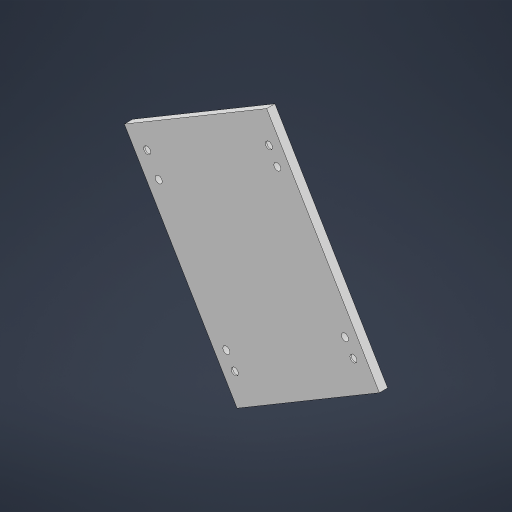
# Autodesk Inventor part: ThirdPlate
Saved by Autodesk Inventor 2024.2 (Build 282272000, 272)
## iProperties
Created: 2023-12-27
Part Number: ThirdPlate
Material: 一般
Document SubType Name: Modeling
Designer: Hanaoka
Density: 1 g/cm^3
Appearance: 既定
Author: Hanaoka
Autodesk Inventor part; units mm, degrees
ref_plane "YZ Plane" through (0, 0, 0) normal (1, 0, 0) x (0, 1, 0)
ref_plane "XZ Plane" through (0, 0, 0) normal (0, 1, 0) x (-1, 0, 0)
ref_plane "XY Plane" through (0, 0, 0) normal (0, 0, 1) x (1, 0, 0)
sketch "スケッチ1" plane through (0, 0, 0) normal (0, 0, 1) x (1, 0, 0)
  line L0 (9.406, -6.0438) -> (-42.1785, -36.6875)
  line L1 (-42.1785, -36.6875) -> (-83.0369, 32.0918)
  line L2 (-83.0369, 32.0918) -> (-31.4524, 62.7355)
  line L3 (-31.4524, 62.7355) -> (9.406, -6.0438)
  circle A0 centre (-42.9871, -25.5365) radius 1.3 projected
  circle A1 centre (-74.7819, 27.9857) radius 1.3 projected
  circle A2 centre (-30.6438, 51.5845) radius 1.3 projected
  circle A3 centre (0, 0) radius 1.3 projected
  line L4 (-30.6438, 51.5845) -> (-26.3451, 54.1381) construction
  line L5 (-30.6438, 51.5845) -> (-35.7511, 60.1819) construction
  line L6 (-42.9871, -25.5365) -> (-47.2858, -28.0901) construction
  line L7 (-42.9871, -25.5365) -> (-37.8798, -34.1339) construction
  line L8 (-74.7819, 27.9857) -> (-78.7381, 34.6454) construction
  line L9 (-74.7819, 27.9857) -> (-79.0806, 25.432) construction
  line L10 (0, 0) -> (4.2987, 2.5536) construction
  line L11 (0, 0) -> (5.1073, -8.5974) construction
  circle A4 centre (0, 0) radius 2.5
  circle A5 centre (-74.7819, 27.9857) radius 2.5
  circle A6 centre (-42.9871, -25.5365) radius 2.5
  circle A7 centre (-30.6438, 51.5845) radius 2.5
  line L12 (-6.6841, 48.3706) -> (8.6378, 22.5784)
  line L13 (8.6378, 22.5784) -> (0.7535, 8.5216)
  line L14 (-74.3843, 17.5264) -> (-82.2686, 3.4696)
  line L15 (-82.2686, 3.4696) -> (-66.9467, -22.3226)
  line L16 (-66.9467, -22.3226) -> (-50.831, -22.1222)
  line L17 (-6.6841, 48.3706) -> (-22.7998, 48.1702)
  line L18 (-74.6077, -9.4265) -> (0.9768, 35.4745) construction
  line L19 (-11.0232, 28.3459) -> (0.9768, 35.4745) construction
  line L20 (-62.6077, -2.2979) -> (-74.6077, -9.4265) construction
  point P0 (0, 0)
  dimension "d2" = 80
  dimension "d3" = 60
  dimension "d4" = 5
  dimension "d13" = 30
  dimension "d15" = 120
  dimension "d16" = 12
  constraints: 42 end point, 14 point on line, 9 perpendicular, 8 equal length, 5 midpoint, 5 parallel, 4 centre point, 4 coincident, 3 equal radius
  measures "d2" distance of L2.end L0.start
  measures "d3" distance of L1.end L2.end
  measures "d4" diameter of A7
  measures "d13" distance of L14.end L15.end
  measures "d15" angle of L12 L17
  measures "d16" horizontal distance of L18.end L19.start
extrude "押し出し1" add sketch "スケッチ1" along normal blind 0.5 contours L0 L1 L2 L3 | A4 | A5 | A6 | A7
sketch "スケッチ2" plane through (0, 0, 0) normal (0, 0, -1) x (-1, 0, 0)
  circle A0 centre (0, 0) radius 2.55
  circle A1 centre (42.9871, -25.5365) radius 1.3 projected
  circle A2 centre (42.9871, -25.5365) radius 2.55
  circle A3 centre (74.7819, 27.9857) radius 1.3 projected
  circle A4 centre (74.7819, 27.9857) radius 2.55
  circle A5 centre (30.6438, 51.5845) radius 1.3 projected
  circle A6 centre (30.6438, 51.5845) radius 2.55
  line L0 (31.4524, 62.7355) -> (83.0369, 32.0918) projected
  line L1 (-9.406, -6.0438) -> (31.4524, 62.7355) projected
  line L2 (42.1785, -36.6875) -> (-9.406, -6.0438) projected
  line L3 (83.0369, 32.0918) -> (42.1785, -36.6875) projected
  circle A7 centre (0, 0) radius 1.3 projected
  circle A8 centre (30.6438, 51.5845) radius 1.3 projected
  circle A9 centre (74.7819, 27.9857) radius 1.3 projected
  circle A10 centre (42.9871, -25.5365) radius 1.3 projected
  dimension "d5" = 5.1
  constraints: 4 centre point, 4 coincident, 3 equal radius
  measures "d5" diameter of A2
extrude "押し出し2" add sketch "スケッチ2" along normal blind 2.5 contours L0 L3 L2 L1
sketch "スケッチ3" plane through (0, 0, 0.5) normal (0, 0, 1) x (1, 0, 0)
  line L0 (-46.0514, -20.378) -> (-70.5665, 20.8896) construction
  line L1 (-70.5665, 20.8896) -> (-27.5794, 46.426) construction
  line L2 (-27.5794, 46.426) -> (-3.0644, 5.1584) construction
  line L3 (-3.0644, 5.1584) -> (-46.0514, -20.378) construction
  line L4 (-31.4524, 62.7355) -> (-83.0369, 32.0918) projected
  line L5 (-83.0369, 32.0918) -> (-42.1785, -36.6875) projected
  line L6 (-42.1785, -36.6875) -> (9.406, -6.0438) projected
  line L7 (9.406, -6.0438) -> (-31.4524, 62.7355) projected
  circle A0 centre (0, 0) radius 1.3 projected
  circle A1 centre (-30.6438, 51.5845) radius 1.3 projected
  circle A2 centre (-74.7819, 27.9857) radius 1.3 projected
  circle A3 centre (-42.9871, -25.5365) radius 1.3 projected
  line L8 (-83.0369, 32.0918) -> (-42.1785, -36.6875) projected
  line L9 (-31.4524, 62.7355) -> (-83.0369, 32.0918) projected
  line L10 (-62.6077, -2.2979) -> (-11.0232, 28.3459) construction
  line L11 (-16.3862, -21.3657) -> (-57.2446, 47.4137) construction
  line L12 (-70.5665, 20.8896) -> (-3.0644, 5.1584) construction
  line L13 (-46.0514, -20.378) -> (-27.5794, 46.426) construction
  circle A4 centre (-70.5665, 20.8896) radius 1.3
  circle A5 centre (-46.0514, -20.378) radius 1.3
  circle A6 centre (-27.5794, 46.426) radius 1.3
  circle A7 centre (-3.0644, 5.1584) radius 1.3
  point P0 (0, 0)
  point P1 (-36.8154, 13.024)
  point P2 (-36.8154, 13.024)
  point P3 (-36.8154, 13.024)
  point P4 (-36.8154, 13.024)
  point P5 (-36.8154, 13.024)
  dimension "d8" = 48
  dimension "d9" = 50
  dimension "d10" = 2.6
  constraints: 16 end point, 8 midpoint, 5 coincident, 4 centre point, 3 equal radius, 3 parallel, 3 point on line, 1 perpendicular
  measures "d8" distance of L0.start L0.end
  measures "d9" distance of L0.end L1.end
  measures "d10" diameter of A4
extrude "押し出し3" cut sketch "スケッチ3" against normal up to surface (3 mm away) contours A4 | A5 | A6 | A7
